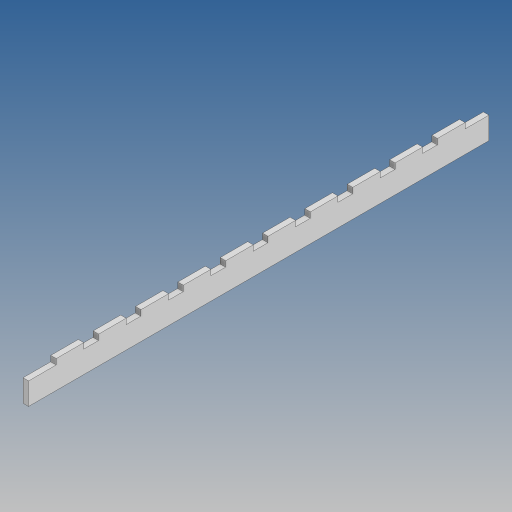
# Autodesk Inventor part: Pieza2
Saved by Autodesk Inventor 2024 (Build 280153000, 153)
## iProperties
Created: 2024-05-31
Part Number: Pieza2
Material: Genérico
Document SubType Name: Modeling
Designer: Pablo
Density: 1 g/cm^3
Appearance: Valor por defecto
Author: Pablo
Autodesk Inventor part; units mm, degrees
ref_plane "YZ Plane" through (0, 0, 0) normal (1, 0, 0) x (0, 1, 0)
ref_plane "XZ Plane" through (0, 0, 0) normal (0, 1, 0) x (-1, 0, 0)
ref_plane "XY Plane" through (0, 0, 0) normal (0, 0, 1) x (1, 0, 0)
sketch "Boceto1" plane through (0, 0, 0) normal (1, 0, 0) x (0, 1, 0)
  line L0 (0, 0) -> (12, 0)
  line L1 (12, 0) -> (12, -250)
  line L2 (12, -250) -> (0, -250)
  line L3 (0, -250) -> (0, 0)
  line L4 (12, -15) -> (12, -30)
  line L5 (12, -30) -> (15, -30)
  line L6 (15, -30) -> (15, -15)
  line L7 (15, -15) -> (12, -15)
  line L8 (15, -53) -> (15, -38)
  line L9 (15, -38) -> (12, -38)
  line L10 (12, -38) -> (12, -53)
  line L11 (12, -53) -> (15, -53)
  line L12 (15, -76) -> (15, -61)
  line L13 (15, -61) -> (12, -61)
  line L14 (12, -61) -> (12, -76)
  line L15 (12, -76) -> (15, -76)
  line L16 (15, -99) -> (15, -84)
  line L17 (15, -84) -> (12, -84)
  line L18 (12, -84) -> (12, -99)
  line L19 (12, -99) -> (15, -99)
  line L20 (15, -122) -> (15, -107)
  line L21 (15, -107) -> (12, -107)
  line L22 (12, -107) -> (12, -122)
  line L23 (12, -122) -> (15, -122)
  line L24 (15, -145) -> (15, -130)
  line L25 (15, -130) -> (12, -130)
  line L26 (12, -130) -> (12, -145)
  line L27 (12, -145) -> (15, -145)
  line L28 (15, -168) -> (15, -153)
  line L29 (15, -153) -> (12, -153)
  line L30 (12, -153) -> (12, -168)
  line L31 (12, -168) -> (15, -168)
  line L32 (15, -191) -> (15, -176)
  line L33 (15, -176) -> (12, -176)
  line L34 (12, -176) -> (12, -191)
  line L35 (12, -191) -> (15, -191)
  line L36 (15, -214) -> (15, -199)
  line L37 (15, -199) -> (12, -199)
  line L38 (12, -199) -> (12, -214)
  line L39 (12, -214) -> (15, -214)
  line L40 (15, -237) -> (15, -222)
  line L41 (15, -222) -> (12, -222)
  line L42 (12, -222) -> (12, -237)
  line L43 (12, -237) -> (15, -237)
  point P0 (12, -128)
  point P1 (13.5, -15)
  point P2 (13.5, -38)
  point P3 (13.5, -61)
  point P4 (13.5, -84)
  point P5 (13.5, -107)
  point P6 (13.5, -130)
  point P7 (13.5, -153)
  point P8 (13.5, -176)
  point P9 (13.5, -199)
  point P10 (13.5, -222)
  point P11 (12, -107)
  point P12 (12, -99)
  point P13 (12, -84)
  point P14 (12, -76)
  point P15 (12, -61)
  point P16 (12, -53)
  point P17 (12, -38)
  point P18 (12, -30)
  point P19 (12, -15)
  point P20 (12, -237)
  point P21 (12, -222)
  point P22 (12, -214)
  point P23 (12, -199)
  point P24 (12, -191)
  point P25 (12, -176)
  point P26 (12, -168)
  point P27 (12, -153)
  point P28 (12, -145)
  point P29 (12, -130)
  point P30 (12, -122)
  dimension "d0" = 12
  dimension "d1" = 250
  dimension "d2" = 15
  dimension "d3" = 3
  dimension "d4" = 23
  constraints: 86 end point, 3 parallel, 2 horizontal, 1 midpoint, 1 perpendicular, 1 vertical, 3 other
  measures "d0" distance of L2.start L2.end
  measures "d1" distance of L0.end L2.start
  measures "d2" distance of L6.end L5.end
  measures "d3" distance of L5.end L5.start
  measures "d4" distance of L6.end L8.end
extrude "Extrusión1" add sketch "Boceto1" along normal blind 3
